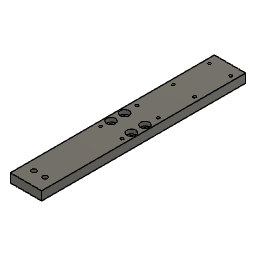
Z-AxisGearRackPlateFixed v11 (Autodesk Fusion 360 archive; units mm, degrees)
design "Z-AxisGearRackPlateFixed" references "tormach 770mx"
Autodesk Fusion 360 part; units mm, degrees
sketch "Sketch1" plane through (0, 0, 0) normal (0, 1, 0) x (1, 0, 0)
  line L0 (0, 0) -> (23, 0)
  line L1 (23, 0) -> (23, -150)
  line L2 (23, -150) -> (0, -150)
  line L3 (0, -150) -> (0, 0)
  dimension "d1" = 23
  dimension "d2" = 150
  constraint horizontal L0
  constraint vertical L1
  constraint horizontal L2
  constraint vertical L3
  constraint coincident L0.start L3.end
  measures "d1" distance of L0.start L0.end
  measures "d2" distance of L0.start L2.end
extrude "Extrude1" add sketch "Sketch1" along normal blind 6.43
sketch "Sketch2" plane through (0, 6.43, 0) normal (0, 1, 0) x (1, 0, 0)
  line L0 (11.5, 0) -> (11.5, -150) construction
  line L1 (0, 0) -> (0, -150)
  line L2 (0, -75) -> (23, -75) construction
  line L3 (19, -70) -> (4, -70) construction
  line L4 (4, -70) -> (4, -80) construction
  line L5 (4, -80) -> (19, -80) construction
  line L6 (19, -80) -> (19, -70) construction
  line L7 (19, -70) -> (4, -80) construction
  line L8 (4, -70) -> (19, -80) construction
  line L9 (23, 0) -> (0, 0)
  line L10 (0, -150) -> (23, -150)
  line L11 (0, -150) -> (23, -150)
  line L12 (23, -150) -> (23, 0)
  line L13 (23, 0) -> (0, 0)
  line L14 (0, 0) -> (0, -150)
  point P0 (11.5, -75)
  point P1 (4, -70)
  point P2 (19, -70)
  point P3 (19, -80)
  point P4 (4, -80)
  point P5 (3.7, -7.25)
  point P6 (19.3, -7.25)
  point P7 (3.7, -33.92)
  point P8 (3.7, -60.59)
  point P9 (3.7, -87.26)
  point P10 (19.3, -33.92)
  point P11 (19.3, -60.59)
  point P12 (19.3, -87.26)
  dimension "d5" = 11.5
  dimension "d6" = 15
  dimension "d7" = 10
  dimension "d8" = 15.6
  dimension "d9" = 19.3
  dimension "d10" = 7.25
  dimension "d13" = 0
  dimension "d14" = -26.67
  dimension "d17" = 0
  dimension "d18" = -26.67
  constraint vertical L0
  constraint midpoint L1 L2.start
  constraint perpendicular L0 L2
  constraint horizontal L3
  constraint perpendicular L3 L4
  constraint parallel L3 L5
  constraint parallel L4 L6
  constraint coincident L7 P0
  constraint coincident L8 P0
  constraint midpoint L0 P0
  constraint coincident P1 L3.end
  constraint coincident P2 L3.start
  constraint coincident P3 L5.end
  constraint coincident P4 L4.end
  constraint horizontal P5 P6
  measures "d5" distance of L0 L1
  measures "d6" distance of P4 P3
  measures "d7" distance of P1 P4
  measures "d8" distance of P5 P6
  measures "d9" distance of L1 P6
  measures "d10" distance of P5 L9
hole "Hole1" at (4, 6.43, 70) direction (0, -1, 0) diameter 3.4 end through all counterbore diameter 6.5 counterbore depth 3
hole "Hole2" at (19, 6.43, 70) direction (0, -1, 0) diameter 3.4 end through all counterbore diameter 6.5 counterbore depth 3
hole "Hole3" at (4, 6.43, 80) direction (0, -1, 0) diameter 3.4 end through all counterbore diameter 6.5 counterbore depth 3
hole "Hole4" at (19, 6.43, 80) direction (0, -1, 0) diameter 3.4 end through all counterbore diameter 6.5 counterbore depth 3
hole "Hole5" at (3.7, 6.43, 7.25) direction (0, -1, 0) diameter 2.05 end through all
hole "Hole6" at (19.3, 6.43, 7.25) direction (0, -1, 0) diameter 2.05 end through all
hole "Hole7" at (3.7, 6.43, 33.92) direction (0, -1, 0) diameter 2.05 end through all
hole "Hole8" at (19.3, 6.43, 33.92) direction (0, -1, 0) diameter 2.05 end through all
hole "Hole9" at (3.7, 6.43, 60.59) direction (0, -1, 0) diameter 2.05 end through all
hole "Hole10" at (19.3, 6.43, 60.59) direction (0, -1, 0) diameter 2.05 end through all
hole "Hole11" at (3.7, 6.43, 87.26) direction (0, -1, 0) diameter 2.05 end through all
hole "Hole12" at (19.3, 6.43, 87.26) direction (0, -1, 0) diameter 2.05 end through all
sketch "Sketch3" plane through (0, 0, 0) normal (0, -1, 0) x (1, 0, 0)
  circle A0 centre (19.3, 87.26) radius 1.025
  circle A1 centre (3.7, 87.26) radius 1.025
  circle A2 centre (19.3, 60.59) radius 1.025
  circle A3 centre (3.7, 60.59) radius 1.025
  circle A4 centre (19.3, 33.92) radius 1.025
  circle A5 centre (3.7, 33.92) radius 1.025
  circle A6 centre (19.3, 7.25) radius 1.025
  circle A7 centre (3.7, 7.25) radius 1.025
  circle A8 centre (19, 80) radius 1.7
  circle A9 centre (4, 80) radius 1.7
  circle A10 centre (19, 70) radius 1.7
  circle A11 centre (4, 70) radius 1.7
  line L0 (23, 150) -> (0, 150)
  line L1 (0, 150) -> (0, 0)
  line L2 (0, 0) -> (23, 0)
  line L3 (23, 0) -> (23, 150)
  line L4 (0, 150) -> (23, 150)
  point P0 (15.6, 140)
  point P1 (7.46, 140)
  dimension "d92" = 8.14
  dimension "d93" = 10
  dimension "d94" = 7.4
  constraint horizontal P0 P1
  measures "d92" distance of P0 P1
  measures "d93" distance of P0 L4
  measures "d94" distance of L3 P0
hole "Hole17" at (7.4, 0, 140) direction (0, 1, 0) diameter 3.4 end through all counterbore diameter 6.5 counterbore depth 3
hole "Hole18" at (15.54, 0, 140) direction (0, 1, 0) diameter 3.4 end through all counterbore diameter 6.5 counterbore depth 3
